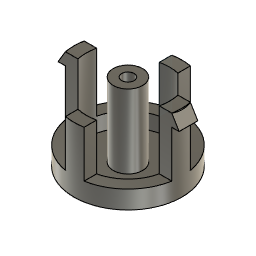
power-button (Autodesk Fusion 360 design; units mm, degrees)
Autodesk Fusion 360 part; units mm, degrees
sketch "Base" plane through (0, 0, 0) normal (0, 0, 1) x (1, 0, 0)
  circle A0 centre (15, 15) radius 11
  dimension "d1" = 22
  measures "d1" diameter of A0
  measures "d5" diameter of A0.centre
extrude "Extrude1" add sketch "Base" along normal blind 18
sketch "Towers" plane through (0, 0, 18) normal (0, 0, 1) x (-1, 0, 0)
  circle A0 centre (-15, -15) radius 11
  line L0 (-15, -15) -> (-26, -15)
  line L1 (-15, -15) -> (-15, -26)
  line L2 (-15, -15) -> (-4, -15)
  line L3 (-15, -15) -> (-15, -4)
  circle A1 centre (-15, -15) radius 3
  circle A2 centre (-15, -15) radius 8.5
  line L4 (-13.1, -25.8347) -> (-13.1, -23.2849)
  line L5 (-16.9, -25.8347) -> (-16.9, -23.2849)
  line L6 (-4.1653, -16.9) -> (-6.7151, -16.9)
  line L7 (-4.1653, -13.1) -> (-6.7151, -13.1)
  line L8 (-23.2849, -16.9) -> (-25.8347, -16.9)
  line L9 (-23.2849, -13.1) -> (-25.8347, -13.1)
  line L10 (-13.1, -6.7151) -> (-13.1, -4.1653)
  line L11 (-16.9, -6.7151) -> (-16.9, -4.1653)
  circle A3 centre (-15, -15) radius 1.27
  dimension "d4" = 6
  dimension "d5" = 17
  dimension "d6" = 1.9
  dimension "d7" = 1.9
  dimension "d8" = 1.9
  dimension "d9" = 1.9
  dimension "d10" = 1.9
  dimension "d11" = 1.9
  dimension "d12" = 1.9
  dimension "d13" = 1.9
  dimension "d14" = 2.54
  constraint coincident A0.centre L0.start
  constraint coincident A0 L0.end
  constraint horizontal L0
  constraint coincident A0 L1.end
  constraint perpendicular L0 L1
  constraint coincident A0 L2.end
  constraint perpendicular L1 L2
  constraint coincident A0 L3.end
  constraint perpendicular L0 L3
  constraint coincident A0 L4.start
  constraint coincident A2 L4.end
  constraint vertical L4
  constraint coincident A0 L5.start
  constraint coincident A2 L5.end
  constraint parallel L4 L5
  constraint coincident A0 L6.start
  constraint coincident A2 L6.end
  constraint horizontal L6
  constraint coincident A0 L7.start
  constraint coincident A2 L7.end
  constraint parallel L2 L7
  constraint coincident A2 L8.start
  constraint coincident A0 L8.end
  constraint parallel L0 L8
  constraint coincident A2 L9.start
  constraint coincident A0 L9.end
  constraint parallel L0 L9
  constraint coincident A2 L10.start
  constraint coincident A0 L10.end
  constraint perpendicular L2 L10
  constraint coincident A2 L11.start
  constraint coincident A0 L11.end
  constraint parallel L3 L11
  measures "d4" diameter of A1
  measures "d5" diameter of A2
  measures "d6" distance of L1 L5
  measures "d7" distance of L1 L4
  measures "d8" distance of L2 L6
  measures "d9" distance of L2 L7
  measures "d10" distance of L0 L8
  measures "d11" distance of L0 L9
  measures "d12" distance of L3 L10
  measures "d13" distance of L3 L11
  measures "d14" diameter of A3
extrude "Extrude2" cut sketch "Towers" against normal blind 12 contours A0 A2 L7 L10 | A0 A2 L4 L6 | A0 A2 L9 L11 | A0 A2 L5 L8
extrude "Extrude3" cut sketch "Towers" against normal blind 15 contours L1 L2 A1 A2 | L2 L3 A1 A2 | L0 L3 A1 A2 | L0 L1 A1 A2
extrude "Extrude4" cut sketch "Towers" against normal blind 15 contours L1 L2 A3 | L2 L3 A3 | L0 L1 A3 | L0 L3 A3
extrude "Extrude5" cut sketch "Towers" against normal blind 2.5 contours A0 L3 A2 L10 | A0 L1 A2 L4 | A0 L3 A2 L11 | A0 L1 A2 L5
sketch "Hook Left" plane through (0, 13.1, 0) normal (0, -1, 0) x (1, 0, 0)
  line L0 (6.7151, 18) -> (4.1653, 18)
  line L1 (4.1653, 18) -> (4.1653, 6)
  line L2 (4.1653, 6) -> (6.7151, 6)
  line L3 (6.7151, 6) -> (6.7151, 18)
  line L4 (4.1653, 18) -> (2.6653, 15.5)
  line L5 (2.6653, 15.5) -> (4.1653, 15.5)
  dimension "d23" = 2.5
  dimension "d24" = 1.5
  constraint coincident L0.end L1.start
  constraint coincident L1 L5.end
  constraint perpendicular L1 L5
  measures "d23" distance of L0.end L5.end
  measures "d24" distance of L4.end L5.end
extrude "Extrude6" add sketch "Hook Left" against normal blind 3.8 contours L1 L4 L5
sketch "Hook Right" plane through (0, 13.1, 0) normal (0, -1, 0) x (1, 0, 0)
  line L0 (25.8347, 18) -> (23.2849, 18)
  line L1 (23.2849, 18) -> (23.2849, 6)
  line L2 (23.2849, 6) -> (25.8347, 6)
  line L3 (25.8347, 6) -> (25.8347, 18)
  line L4 (25.8347, 18) -> (27.3347, 15.5)
  line L5 (27.3347, 15.5) -> (25.8347, 15.5)
  dimension "d27" = 1.5
  dimension "d28" = 2.5
  constraint coincident L0.start L3.end
  constraint coincident L3 L5.end
  constraint perpendicular L3 L5
  measures "d27" distance of L4.end L5.end
  measures "d28" distance of L0.start L5.end
extrude "Extrude7" add sketch "Hook Right" against normal blind 3.8 contours L3 L4 L5
sketch "Sketch8" plane through (13.1, 0, 0) normal (-1, 0, 0) x (0, -1, 0)
  line L0 (-23.2849, 15.5) -> (-25.8347, 15.5)
  line L1 (-25.8347, 15.5) -> (-25.8347, 6)
  line L2 (-25.8347, 6) -> (-23.2849, 6)
  line L3 (-23.2849, 6) -> (-23.2849, 15.5)
sketch "Curved Top" plane through (0, 0, 0) normal (0, 1, 0) x (1, 0, 0)
  line L0 (15, 0, 15) -> (26.25, 0, 15)
  line L1 (26.25, 0, 15) -> (26.25, -2.5, 15)
  line L2 (26.25, -2.5, 15) -> (15, -2.5, 15)
  line L3 (15, -2.5, 15) -> (15, 0, 15)
  spline S0 degree 5 poles (15, 0, 15) (15.5369, -0.0008, 15) (16.5888, -0.0165, 15) (18.1008, -0.0816, 15) (19.9827, -0.2534, 15) (22.0954, -0.6201, 15) (23.9431, -1.1547, 15) (25.4969, -1.8756, 15) (26.731, -2.799, 15) (27.638, -3.9297, 15) (28.2334, -5.2579, 15) (28.4766, -6.4682, 15) (28.5356, -7.4542, 15) (28.5209, -8.1457, 15) (28.5, -8.5, 15) knots 0 0 0 0 0 0 0.1 0.2 0.3 0.4 0.5 0.6 0.7 0.8 0.9 1 1 1 1 1 1
revolve "Revolve5" cut sketch "Curved Top" angle 360 about axis through (15, 15, 2.5) along (0, 0, -1) contours L0 L1 S0 in plane through (0, 15, 0) normal (0, 1, 0)
revolve "Revolve4" [rolled back] along angle 360
equation "d5 = ( 8.5 * 2 ) * 1 mm"
equation "d6 = 3.8 mm / 2"
equation "d7 = ( 3.8 / 2 ) * 1 mm"
equation "d8 = ( 3.80 / 2 ) * 1 mm"
equation "d9 = ( 3.8 / 2 ) * 1 mm"
equation "d10 = ( 3.8 / 2 ) * 1 mm"
equation "d11 = ( 3.8 / 2 ) * 1 mm"
equation "d12 = ( 3.8 / 2 ) * 1 mm"
equation "d13 = ( 3.8 / 2 ) * 1 mm"
equation "d15 = -18.00 mm + 6 mm"
equation "d17 = -18 mm + 3 mm"
equation "d19 = -18 mm + 3 mm"
named bodies: "Power Button"
